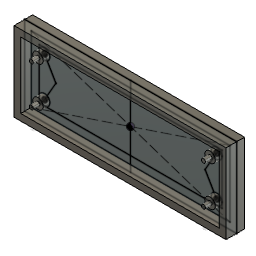
uFluidic-Model-Base v0 (Autodesk Fusion 360 design; units mm, degrees)
Autodesk Fusion 360 part; units mm, degrees
note: some values were not read from the file. Set by a fixed rule: which sketch regions a step uses.
sketch "Sketch1" plane through (0, 0, 0) normal (0, 0, 1) x (1, 0, 0)
  line L0 (37.5, 12.5) -> (-37.5, 12.5)
  line L1 (-37.5, 12.5) -> (-37.5, -12.5)
  line L2 (-37.5, -12.5) -> (37.5, -12.5)
  line L3 (37.5, -12.5) -> (37.5, 12.5)
  line L4 (37.5, 12.5) -> (-37.5, -12.5) construction
  line L5 (-37.5, 12.5) -> (37.5, -12.5) construction
  line L6 (-40, -15) -> (40, -15)
  line L7 (40, -15) -> (40, 15)
  line L8 (40, 15) -> (-40, 15)
  line L9 (-40, 15) -> (-40, -15)
  line L10 (-34.5, -9.5) -> (34.5, -9.5)
  line L11 (34.5, -9.5) -> (34.5, 9.5)
  line L12 (34.5, 9.5) -> (-34.5, 9.5)
  line L13 (-34.5, 9.5) -> (-34.5, -9.5)
  line L14 (0, 15) -> (0, -15)
  circle A0 centre (-32.5, 7.5) radius 0.75
  circle A1 centre (-32.5, 7.5) radius 2
  circle A2 centre (-32.5, -7.5) radius 2
  circle A3 centre (-32.5, -7.5) radius 0.75
  circle A4 centre (32.5, -7.5) radius 0.75
  circle A5 centre (32.5, -7.5) radius 2
  circle A6 centre (32.5, 7.5) radius 0.75
  circle A7 centre (32.5, 7.5) radius 2
  line L15 (-32.5, 7.5) -> (-28.1699, 0)
  line L16 (-28.1699, 0) -> (-32.5, -7.5)
  line L17 (32.5, -7.5) -> (28.1699, 0)
  line L18 (28.1699, 0) -> (32.5, 7.5)
  dimension "d1" = 75
  dimension "d2" = 25
  dimension "d3" = 2.5
  dimension "d4" = -3
  dimension "d5" = 1.5
  dimension "d6" = 4
  dimension "d7" = 4
  dimension "d8" = 1.5
  dimension "d9" = 1.5
  dimension "d10" = 4
  dimension "d11" = 1.5
  dimension "d12" = 4
  dimension "d16" = 30
  dimension "d17" = 30
  dimension "d18" = 30
  dimension "d19" = 30
  constraint horizontal L0
  constraint perpendicular L0 L1
  constraint parallel L0 L2
  constraint parallel L1 L3
  constraint coincident L4 origin
  constraint coincident L5 origin
  constraint midpoint L8 L14.start
  constraint midpoint L6 L14.end
  constraint concentric A0 A1
  constraint tangent L12 A1
  constraint tangent L13 A1
  constraint concentric A2 A3
  constraint tangent L10 A2
  constraint tangent L13 A2
  constraint concentric A4 A5
  constraint tangent L11 A5
  constraint tangent L10 A5
  constraint concentric A6 A7
  constraint tangent L11 A7
  constraint tangent L12 A7
  constraint coincident A0.centre A1.centre
  constraint coincident A2.centre A3.centre
  constraint coincident A4.centre A5.centre
  constraint coincident A6.centre A7.centre
  measures "d1" distance of L1.end L2.end
  measures "d2" distance of L0.end L1.end
  measures "d5" diameter of A0
  measures "d6" diameter of A1
  measures "d7" diameter of A2
  measures "d8" diameter of A3
  measures "d9" diameter of A4
  measures "d10" diameter of A5
  measures "d11" diameter of A6
  measures "d12" diameter of A7
  measures "d16" angle of L13 L15
  measures "d17" angle of L13 L16
  measures "d18" angle of L11 L18
  measures "d19" angle of L11 L17
extrude "Extrude1" add sketch "Sketch1" against normal blind 3 contours L0 L2 L3 L10 L11 L12 L14 | L0 L2 L3 L6 L7 L8 L14 | L0 L1 L2 L10 L12 L13 L14 | L0 L1 L2 L6 L8 L9 L14 | L10 L12 L14 A1 A2 L15 L16 | L10 L12 L14 A5 A7 L17 L18 | L11 L12 A7 | A7 | L12 L13 A1 | A1 | L11 A5 A7 L17 L18 | L13 A1 A2 L15 L16 | L10 L13 A2 | A2 | L10 L11 A5 | A5 | A0 | A3 | A4 | A6
extrude "Extrude2" add sketch "Sketch1" along normal blind 4 contours L0 L2 L3 L6 L7 L8 L14 | L0 L1 L2 L6 L8 L9 L14
extrude "Extrude3" add sketch "Sketch1" along normal blind 2.5 contours A7 | A1 | A2 | A5 | A0 | A3 | A4 | A6
extrude "Extrude5" add sketch "Sketch1" along normal blind 5 contours A0 | A3 | A4 | A6
